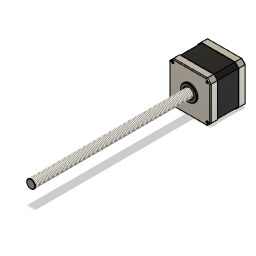
Stepper Motor Through Hole v1 (Autodesk Fusion 360 design; units mm, degrees)
Autodesk Fusion 360 part; units mm, degrees
sketch "Skizze1" plane through (0, 0, 0) normal (0, 0, 1) x (1, 0, 0)
  line L0 (-28, 28) -> (28, 28)
  line L1 (28, 28) -> (28, -28)
  line L2 (28, -28) -> (-28, -28)
  line L3 (-28, -28) -> (-28, 28)
  line L4 (28, 0) -> (-28, 0) construction
  line L5 (0, 28) -> (0, -28) construction
  line L6 (-23.5, 23.5) -> (23.5, 23.5) construction
  line L7 (23.5, 23.5) -> (23.5, -23.5) construction
  line L8 (23.5, -23.5) -> (-23.5, -23.5) construction
  line L9 (-23.5, -23.5) -> (-23.5, 23.5) construction
  line L10 (0, 23.5) -> (0, -23.5) construction
  line L11 (-23.5, 0) -> (23.5, 0) construction
  circle A0 centre (0, 0) radius 11
  circle A1 centre (0, 0) radius 6
  circle A2 centre (0, 0) radius 7.5
  point P0 (23.5, 23.5)
  point P1 (23.5, -23.5)
  point P2 (-23.5, -23.5)
  point P3 (-23.5, 23.5)
  dimension "d1" = 56
  dimension "d2" = 56
  dimension "d3" = 47
  dimension "d4" = 47
  dimension "d5" = 22
  dimension "d9" = 12
  dimension "d22" = 15
  constraint horizontal L0
  constraint vertical L1
  constraint horizontal L2
  constraint vertical L3
  constraint midpoint L1 L4.start
  constraint midpoint L3 L4.end
  constraint midpoint L0 L5.start
  constraint midpoint L2 L5.end
  constraint midpoint L4 A0.centre
  constraint coincident A0.centre A1.centre
  constraint horizontal L6
  constraint vertical L7
  constraint horizontal L8
  constraint vertical L9
  constraint midpoint L6 L10.start
  constraint midpoint L8 L10.end
  constraint midpoint L9 L11.start
  constraint midpoint L7 L11.end
  constraint midpoint L11 A0.centre
  constraint coincident P0 L6.end
  constraint coincident P1 L7.end
  constraint coincident P2 L8.end
  constraint coincident P3 L6.start
  measures "d1" distance of L0.start L0.end
  measures "d2" distance of L0.start L2.end
  measures "d3" distance of P3 P0
  measures "d4" distance of P3 P2
  measures "d5" diameter of A0
  measures "d9" diameter of A1
  measures "d22" diameter of A2
extrude "Extrusion1" add sketch "Skizze1" along normal blind 2 contours A0 | A1 | A2 makes body 1
extrude "Extrusion2" add sketch "Skizze1" against normal blind 9.6 separate body contours L0 L1 L2 L3 | A0 | A2 makes body 2
hole "Bohrung1" at (23.5, 23.5, 0) at (-23.5, 23.5, 0) at (-23.5, -23.5, 0) at (23.5, -23.5, 0) direction (0, 0, -1) diameter 2.529 depth 4.5 tip angle 118 countersink diameter 2.782 countersink angle 90 bodies 2
thread "Gewinde1" "ISO Metric profile 3.0 M3x0.5 6H" major diameter 3.086 minor diameter 2.529 pitch 0.5 angle 60 modelled right hand crest width 0.1368 on face at (23.6259, 22.2418, -1.5843) crest through (24.7645, 23.5, -0.2515) on face at (-23.3741, 22.2418, -1.5843) crest through (-22.2355, 23.5, -0.2515) on face at (-23.3741, -24.7582, -1.5843) crest through (-22.2355, -23.5, -0.2515) on face at (23.6259, -24.7582, -1.5843) crest through (24.7645, -23.5, -0.2515) on bodies 2
extrude "Extrusion3" add sketch "Skizze1" along normal blind 215.9 separate body contours A1 makes body 3
chamfer "Fase2" distance 0.5 angle 45 2 edges at (-5.594, -2.1697, 0) (-5.594, -2.1697, 215.9) on bodies 3
extrude "Extrusion4" cut sketch "Skizze1" along normal blind 2 contours A1 | A2 bodies 1
extrude "Extrusion5" add 1 faces at (-0.1495, -20.6611, -9.6) along direction (0, 0, -1) blind 28.8 separate body on bodies 2 makes body 4
extrude "Extrusion6" add 1 faces at (-0.1495, -20.6611, -38.4) along direction (0, 0, -1) blind 9.6 separate body on bodies 4 makes body 5
sketch "Skizze2" plane through (0, 0, -48) normal (0, 0, -1) x (-1, 0, 0)
  circle A0 centre (0, 0) radius 6
  line L0 (-28, -28) -> (28, -28)
  line L1 (28, -28) -> (28, 28)
  line L2 (28, 28) -> (-28, 28)
  line L3 (-28, 28) -> (-28, -28)
  circle A1 centre (0, 0) radius 7.5
extrude "Extrusion7" cut sketch "Skizze2" against normal blind 2 contours A1 bodies 5
chamfer "Fase1" distance 5 angle 45 12 edges at (-28, 28, -24) (28, 28, -24) (28, -28, -24) (-28, -28, -24) (-28, 28, -43.2) (28, 28, -43.2) (28, -28, -43.2) (-28, -28, -43.2) (-28, 28, -4.8) (28, 28, -4.8) (28, -28, -4.8) (-28, -28, -4.8) on bodies 2 4 5
fillet "Abrundung1" radius 1 8 edges at (0, 28, 0) (25.5, 25.5, 0) (28, 0, 0) (25.5, -25.5, 0) (0, -28, 0) (-25.5, -25.5, 0) (-28, 0, 0) (-25.5, 25.5, 0) on bodies 2 5
fillet "Abrundung1" radius 1 8 edges at (0, 28, -48) (25.5, 25.5, -48) (28, 0, -48) (-28, 0, -48) (-25.5, 25.5, -48) (-25.5, -25.5, -48) (0, -28, -48) (25.5, -25.5, -48) on bodies 2 5
fillet "Abrundung2" radius 0.5 1 edges at (-10.2556, -3.9778, 2) on bodies 1
fillet "Abrundung3" radius 0.5 1 edges at (6.9925, 2.7121, -48) on bodies 5
scale "Maßstab1" factors (0.98, 0.98, 1) about (0, 0, 0) bodies 4
thread "Thread2" "ISO Metric profile 12.0 M12x1.75 6g" major diameter 11.8335 minor diameter 9.8365 pitch 1.75 angle 60 resizes the face on face at (5.9925, -0.2991, 143.7667) on bodies 3
equation "d6 = BearingHubSize"
equation "ShaftSize = 5 mm"
equation "Length = 48 mm"
equation "d11 = -CapLength"
equation "CapLength = Length / 5"
equation "d26 = Length - 2 * CapLength"
equation "d28 = CapLength"
equation "BearingHubSize = 2 mm"
equation "FrontHoleDistance = 31 mm" comment "NEMA17: Fixed 31mm"
equation "Width = 42.3 mm" comment "NEMA17 42.0, but we use the max of 42.3mm"
named bodies: "Top cap", "Shaft", "Middle part", "End cap"
